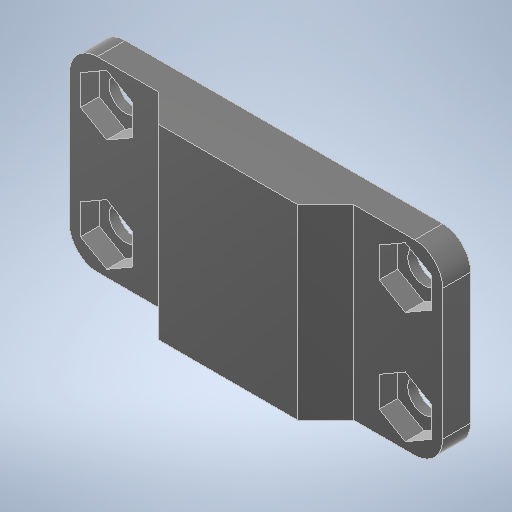
# Autodesk Inventor part: 3D_frame-connect-base1
Saved by Autodesk Inventor 2025 (Build 290162000, 162)
## iProperties
Created: 2024-07-30
Part Number: 3D_frame-connect-base1
Material: 一般
Document SubType Name: Modeling
Designer: 8326d
Density: 1 g/cm^3
Appearance: 滑らか - 黒
Author: 8326d
## iProperties of the stored document 3D_frame-connect-base1_3D プリント.ipt
Created: 2024-08-04
Part Number: 3D_frame-connect-base1_3D プリント
Material: 一般
Document SubType Name: Modeling
Designer: 8326d
Density: 1 g/cm^3
Appearance: 既定
Author: 8326d
Autodesk Inventor part; units mm, degrees
ref_plane "YZ Plane" through (0, 0, 0) normal (1, 0, 0) x (0, 1, 0)
ref_plane "XZ Plane" through (0, 0, 0) normal (0, 1, 0) x (-1, 0, 0)
ref_plane "XY Plane" through (0, 0, 0) normal (0, 0, 1) x (1, 0, 0)
sketch "スケッチ1" plane through (0, 0, 0) normal (0, 0, 1) x (1, 0, 0)
  line L0 (-20, -10) -> (20, -10)
  line L1 (20, -10) -> (20, 10)
  line L2 (20, 10) -> (-20, 10)
  line L3 (-20, 10) -> (-20, -10)
  line L4 (-20, -10) -> (20, 10) construction
  line L5 (20, -10) -> (-20, 10) construction
  point P0 (0, 0)
  dimension "d0" = 40
  dimension "d1" = 20
  constraints: 12 end point, 2 midpoint, 2 parallel, 1 horizontal, 1 perpendicular
  measures "d0" distance of L2.end L1.end
  measures "d1" distance of L1.end L0.end
extrude "押し出し1" add sketch "スケッチ1" along normal blind 3
sketch "スケッチ2" plane through (0, 0, 3) normal (0, 0, 1) x (1, 0, 0)
  line L0 (-16, -6) -> (16, -6) construction
  line L1 (16, -6) -> (16, 6) construction
  line L2 (16, 6) -> (-16, 6) construction
  line L3 (-16, 6) -> (-16, -6) construction
  line L4 (-16, -6) -> (16, 6) construction
  line L5 (16, -6) -> (-16, 6) construction
  point P0 (0, 0)
  dimension "d4" = 32
  dimension "d5" = 12
  constraints: 12 end point, 2 midpoint, 2 parallel, 1 horizontal, 1 perpendicular
  measures "d4" distance of L2.end L1.end
  measures "d5" distance of L1.end L0.end
hole "穴1" at (-16, 6, 3) at (-16, -6, 3) at (16, -6, 3) at (16, 6, 3) direction (0, 0, -1) diameter 3.5 depth 8
sketch "スケッチ3" plane through (0, 0, 3) normal (0, 0, 1) x (1, 0, 0)
  circle A0 centre (-16, 6) radius 1.75 projected
  line L0 (-16, 2.7668) -> (-18.8, 4.3834)
  line L1 (-18.8, 4.3834) -> (-18.8, 7.6166)
  line L2 (-18.8, 7.6166) -> (-16, 9.2332)
  line L3 (-16, 9.2332) -> (-13.2, 7.6166)
  line L4 (-13.2, 7.6166) -> (-13.2, 4.3834)
  line L5 (-13.2, 4.3834) -> (-16, 2.7668)
  point P0 (0, 0)
  point P1 (-21.5, 4.5639)
  point P2 (-21.5, 7.4361)
  dimension "d13" = 5.6
  constraints: 12 end point, 1 coincident, 1 vertical alignment, 14 other
  measures "d13" distance between parallel lines of L1 L4
extrude "押し出し2" cut sketch "スケッチ3" against normal blind 2 contours A0 | L0 L1 L2 L3 L4 L5
pattern_linear "矩形状パターン1" count 2 spacing 32 along (1, 0, 0) count 2 spacing 12 along (0, -1, 0) of "押し出し2"
sketch "スケッチ4" plane through (-20, -10, 0) normal (0, -1, 0) x (1, 0, 0)
  line L0 (0, 3) -> (40, 3) projected
  line L1 (40, 3) -> (0, 3) projected
  line L2 (9.5, 3) -> (12.5, 6)
  line L3 (12.5, 6) -> (27.5, 6)
  line L4 (27.5, 6) -> (30.5, 3)
  line L5 (0, 0) -> (40, 0) projected
  point P0 (20, 0)
  point P1 (20, 6)
  point P2 (20, 0)
  dimension "d22" = 45
  dimension "d23" = 45
  dimension "d24" = 15
  dimension "d25" = 3
  constraints: 6 end point, 2 midpoint, 2 point on line, 1 parallel, 1 vertical alignment
  measures "d22" angle of L0 L2
  measures "d23" angle of L0 L4
  measures "d24" distance of L2.end L3.end
  measures "d25" distance between parallel lines of L0 L3
extrude "押し出し3" add sketch "スケッチ4" against normal up to surface (20 mm away)
fillet "フィレット1" radius 3 4 edges at (-20, 10, 1.5) (-20, -10, 1.5) (20, -10, 1.5) (20, 10, 1.5)
equation "\"d23\" = d22"
